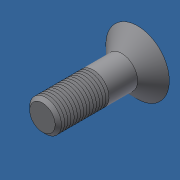
# Autodesk Inventor part: M10x30 Allen Frezato
Saved by Autodesk Inventor 2018 (Build 220112000, 112)
## iProperties
Created: 2016-03-08
Part Number: M10x30 Allen Frezato
Document SubType Name: Modeling
Designer: sakis
Manufacturer: Standard
Standards Organization: Custom
Material: Generic
Density: 1 g/cm^3
Appearance: Default
Author: sakis
Autodesk Inventor part; units mm, degrees
ref_plane "YZ Plane" through (0, 0, 0) normal (1, 0, 0) x (0, 1, 0)
ref_plane "XZ Plane" through (0, 0, 0) normal (0, 1, 0) x (-1, 0, 0)
ref_plane "XY Plane" through (0, 0, 0) normal (0, 0, 1) x (1, 0, 0)
sketch "Sketch1" plane through (0, 0, 0) normal (0, 0, 1) x (1, 0, 0)
  line L0 (0, 19.6828) -> (0, -18.3172)
  line L1 (-0.377, 15.178) -> (-10, 15.178)
  line L2 (-10, 15.178) -> (-5, 10.178)
  line L3 (-5, 10.178) -> (-5, -14.822)
  line L4 (-5, -14.822) -> (0, -14.822)
  line L5 (0, -14.822) -> (0, 15.178)
  line L6 (-0.377, 15.178) -> (0, 15.178)
  dimension "d2" = 20
  dimension "d3" = 45
  dimension "d4" = 30
  dimension "d6" = 10
  constraints: 14 end point, 4 perpendicular, 2 point on line, 1 vertical
  measures "d2" diameter of L1.end L0
  measures "d3" angle of L2 L1
  measures "d4" distance between parallel lines of L1 L4
  measures "d6" diameter of L3 L0
revolve "Revolution1" add sketch "Sketch1" angle 360 about axis through (0, 19.6828, 0) along (0, -1, 0)
chamfer "Chamfer1" distance 1 angle 45 1 edges at (5, -14.822, 0)
sketch "Sketch2" plane through (0, 0, 0) normal (1, 0, 0) x (0, 1, 0)
  line L0 (-13.822, 5) -> (10.178, 5) projected
  line L1 (-13.822, -5) -> (10.178, -5) projected
  line L2 (-13.822, 5) -> (-13.322, 4)
  line L3 (-13.322, 4) -> (-12.822, 5)
  line L4 (-13.822, 5) -> (-12.822, 5)
  line L5 (-12.622, 0) -> (13.978, 0) projected
  dimension "d10" = 1
  dimension "d12" = 1
  constraints: 6 end point, 1 equal length, 1 point on line
  measures "d10" distance from line of L0 L2.end
  measures "d12" distance of L0.start L3.end
revolve "Revolution2" cut sketch "Sketch2" angle 360 about axis through (0, -10, 0) along (0, 1, 0)
pattern_linear "Rectangular Pattern1" count 15 spacing 1 along (0, 1, 0) of "Revolution2"
sketch "Sketch3" plane through (0, 15.178, 0) normal (0, 1, 0) x (1, 0, 0)
  circle A0 centre (0, 0) radius 10 projected
  line L0 (1.7321, -3) -> (-1.7321, -3)
  line L1 (-1.7321, -3) -> (-3.4641, 0)
  line L2 (-3.4641, 0) -> (-1.7321, 3)
  line L3 (-1.7321, 3) -> (1.7321, 3)
  line L4 (1.7321, 3) -> (3.4641, 0)
  line L5 (3.4641, 0) -> (1.7321, -3)
  dimension "d17" = 6
  constraints: 12 end point, 1 coincident, 1 horizontal, 11 other
  measures "d17" distance between parallel lines of L3 L0
extrude "Extrusion1" cut sketch "Sketch3" against normal blind 5 contours L0 L1 L2 L3 L4 L5
body "Solid1"
